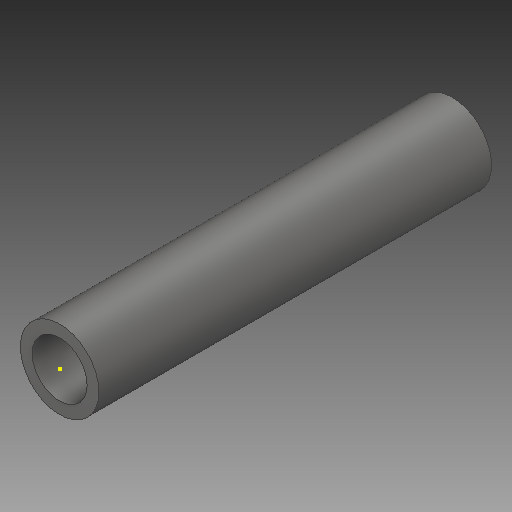
# Autodesk Inventor part: project rolller 1 part
Saved by Autodesk Inventor 2019 (Build 230136000, 136)
## iProperties
Created: 2019-05-14
Part Number: project rolller 1 part
Material: Generic
Document SubType Name: Modeling
Designer: tt1180954
Density: 1 g/cm^3
Appearance: Rubber - Black - Version 1.1
Author: tt1180954
Autodesk Inventor part; units mm, degrees
ref_plane "YZ Plane" through (0, 0, 0) normal (1, 0, 0) x (0, 1, 0)
ref_plane "XZ Plane" through (0, 0, 0) normal (0, 1, 0) x (-1, 0, 0)
ref_plane "XY Plane" through (0, 0, 0) normal (0, 0, 1) x (1, 0, 0)
sketch "Sketch5" plane through (0, 0, 0) normal (0, 0, 1) x (1, 0, 0)
  circle A0 centre (0, 0) radius 50
  dimension "d12" = 100
  constraints: 1 centre point, 1 coincident
  measures "d12" diameter of A0
extrude "Extrusion5" add sketch "Sketch5" along normal blind 500
sketch "Sketch6" plane through (0, 0, 500) normal (0, 0, 1) x (1, 0, 0)
  circle A0 centre (0, 0) radius 35
  dimension "d15" = 70
  constraints: 1 centre point, 1 coincident
  measures "d15" diameter of A0
extrude "Extrusion6" cut sketch "Sketch6" against normal blind 500
sketch "Sketch7" plane through (0, 0, 500) normal (0, 0, 1) x (1, 0, 0)
  point P0 (0, 0)
body "Solid2"
